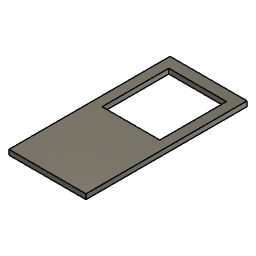
Bauwagen Tür MK1 v3 (Autodesk Fusion 360 design; units mm, degrees)
Autodesk Fusion 360 part; units mm, degrees
sketch "Skizze1" plane through (0, 0, 0) normal (0, 1, 0) x (1, 0, 0)
  line L0 (0, 0) -> (77.5, 0)
  line L1 (77.5, 0) -> (77.5, -162)
  line L2 (77.5, -162) -> (0, -162)
  line L3 (0, -162) -> (0, 0)
  line L4 (0, 0) -> (9.75, 0)
  line L5 (9.75, 0) -> (9.75, -11)
  line L6 (9.75, -11) -> (67.75, -11)
  line L7 (67.75, -11) -> (67.75, -78)
  line L8 (67.75, -78) -> (9.75, -78)
  line L9 (9.75, -78) -> (9.75, -11)
  dimension "d1" = 77.5
  dimension "d2" = 162
  dimension "d3" = 9.75
  dimension "d4" = 11
  dimension "d5" = 67
  dimension "d6" = 58
  constraint coincident L0.start L3.end
  constraint horizontal L0
  constraint perpendicular L0 L1
  constraint perpendicular L1 L2
  constraint perpendicular L0 L3
  constraint perpendicular L3 L4
  constraint perpendicular L4 L5
  constraint horizontal L6
  constraint vertical L7
  constraint horizontal L8
  constraint vertical L9
  measures "d1" distance of L0.start L0.end
  measures "d2" distance of L0.end L1.end
  measures "d3" distance of L0.start L4.end
  measures "d4" distance of L4.end L5.end
  measures "d5" distance of L5.end L8.end
  measures "d6" distance of L5.end L6.end
extrude "Extrusion1" add sketch "Skizze1" along normal blind 5
